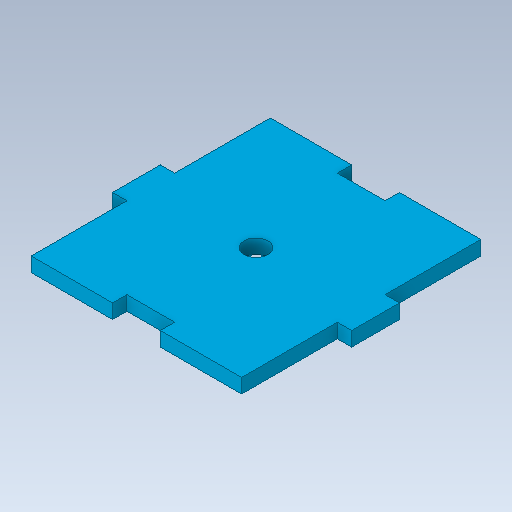
# Autodesk Inventor part: Part8
Saved by Autodesk Inventor 2020 (Build 240168000, 168)
## iProperties
Created: 2020-03-11
Part Number: Part8
Material: Generic
Document SubType Name: Modeling
Designer: tor16003
Density: 1 g/cm^3
Appearance: Sky Blue Medium
Author: tor16003
Autodesk Inventor part; units mm, degrees
ref_plane "YZ Plane" through (0, 0, 0) normal (1, 0, 0) x (0, 1, 0)
ref_plane "XZ Plane" through (0, 0, 0) normal (0, 1, 0) x (-1, 0, 0)
ref_plane "XY Plane" through (0, 0, 0) normal (0, 0, 1) x (1, 0, 0)
sketch "Sketch1" plane through (0, 0, 0) normal (0, 1, 0) x (-1, 0, 0)
  line L0 (0, 0) -> (0, -20)
  line L1 (0, -20) -> (3, -20)
  line L2 (3, -20) -> (3, -30)
  line L3 (3, -30) -> (0, -30)
  line L4 (0, -30) -> (0, -50)
  line L5 (0, -50) -> (-17, -50)
  line L6 (-17, -50) -> (-17, -47)
  line L7 (-17, -47) -> (-27, -47)
  line L8 (-27, -47) -> (-27, -50)
  line L9 (-27, -50) -> (-44, -50)
  line L10 (-44, -50) -> (-44, -30)
  line L11 (-44, -30) -> (-47, -30)
  line L12 (-47, -30) -> (-47, -20)
  line L13 (-47, -20) -> (-44, -20)
  line L14 (-44, -20) -> (-44, 0)
  line L15 (0, 0) -> (-17, 0)
  line L16 (-17, 0) -> (-17, -3)
  line L17 (-17, -3) -> (-27, -3)
  line L18 (-27, -3) -> (-27, 0)
  line L19 (-27, 0) -> (-44, 0)
  circle A0 centre (-22, -25) radius 2.5
  point P0 (3, -25)
  point P1 (-22, -3)
  dimension "d5" = 3
  dimension "d7" = 10
  dimension "d8" = 3
  dimension "d9" = 50
  dimension "d10" = 10
  dimension "d11" = 50
  dimension "d14" = 5
  constraints: 40 end point, 15 perpendicular, 7 equal length, 3 collinear, 3 horizontal, 3 point on line, 2 midpoint, 1 centre point, 1 coincident, 1 horizontal alignment, 1 vertical, 1 vertical alignment
  measures "d5" distance of L7.end L8.end
  measures "d7" distance of L1.end L2.end
  measures "d8" distance of L0.end L1.end
  measures "d9" distance between parallel lines of L12 L2
  measures "d10" distance of L6.end L7.end
  measures "d11" distance between parallel lines of L19 L9
  measures "d14" diameter of A0
extrude "Extrusion2" add sketch "Sketch1" along normal blind 3
body "Solid2"
